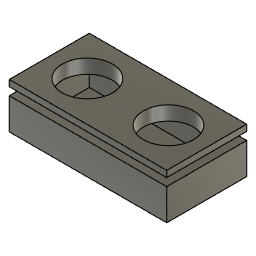
HCSR04 (Autodesk Fusion 360 design; units mm, degrees)
Autodesk Fusion 360 part; units mm, degrees
sketch "top" plane through (0, 0, 0) normal (0, 0, 1) x (1, 0, 0)
  line L0 (22.65, -10.28) -> (-22.65, -10.28)
  line L1 (-22.65, -10.28) -> (-22.65, 10.28)
  line L2 (-22.65, 10.28) -> (22.65, 10.28)
  line L3 (22.65, 10.28) -> (22.65, -10.28)
  line L4 (22.65, -10.28) -> (-22.65, 10.28) construction
  line L5 (-22.65, -10.28) -> (22.65, 10.28) construction
  circle A0 centre (12.95, -0.02) radius 8
  circle A1 centre (-12.95, -0.02) radius 8
  line L6 (-4.95, 0) -> (4.95, 0) construction
  line L7 (-5, -10.28) -> (5, -10.28)
  line L8 (5, -10.28) -> (5, -7.48)
  line L9 (5, -7.48) -> (-5, -7.48)
  line L10 (-5, -7.48) -> (-5, -10.28)
  line L11 (0, -7.48) -> (0, -10.28) construction
  line L12 (25.15, -12.78) -> (-25.15, -12.78)
  line L13 (-25.15, -12.78) -> (-25.15, 12.78)
  line L14 (-25.15, 12.78) -> (25.15, 12.78)
  line L15 (25.15, 12.78) -> (25.15, -12.78)
  line L16 (22.525, -10.155) -> (-22.525, -10.155)
  line L17 (-22.525, -10.155) -> (-22.525, 10.155)
  line L18 (-22.525, 10.155) -> (22.525, 10.155)
  line L19 (22.525, 10.155) -> (22.525, -10.155)
  dimension "d1" = 45.3
  dimension "d2" = 20.56
  dimension "d3" = 16
  dimension "d4" = 16
  dimension "d5" = 2.3
  dimension "d6" = 1.7
  dimension "d7" = 1.7
  dimension "d8" = 2.3
  dimension "d9" = 2.8
  dimension "d10" = 10
  dimension "d11" = -2.5
  dimension "d20" = 0.125
  constraint horizontal L0
  constraint perpendicular L0 L1
  constraint parallel L0 L2
  constraint parallel L1 L3
  constraint coincident L4 origin
  constraint coincident L5 origin
  constraint coincident A1 L6.start
  constraint coincident A0 L6.end
  constraint horizontal L6
  constraint horizontal L7
  constraint vertical L8
  constraint horizontal L9
  constraint vertical L10
  constraint coincident L0 L7.start
  constraint midpoint L9 L11.start
  constraint midpoint L7 L11.end
  constraint midpoint L0 L11.end
  measures "d1" distance of L1.end L2.end
  measures "d2" distance of L0.end L1.end
  measures "d3" diameter of A0
  measures "d4" diameter of A1
  measures "d5" distance of L2 A0
  measures "d6" distance of L3 A0
  measures "d7" distance of L1 A1
  measures "d8" distance of L2 A1
  measures "d9" distance of L7.start L9.end
  measures "d10" distance of L8.end L9.end
extrude "Extrude1" add sketch "top" along normal blind 2 contours L0 L1 L2 L3 L8 L10 L16 L17 L18 L19 | L8 L9 L10 L16 L17 L18 L19 | A0 | A1 | L12 L13 L14 L15 makes body 1
extrude "Extrude2" add sketch "top" along normal blind 8 from surface at 2 contours L12 L13 L14 L15 bodies 1
extrude "Extrude4" add sketch "top" along normal blind 2.5 from surface at 10 separate body contours L8 L9 L10 L16 | L8 L9 L10 L16 L17 L18 L19 makes body 2
extrude "Extrude5" add sketch "top" along normal blind 2 from surface at 12.5 contours L0 L1 L2 L3 L8 L10 L16 L17 L18 L19 | L0 L7 L8 L10 L16 | L8 L9 L10 L16 | L8 L9 L10 L16 L17 L18 L19 | L12 L13 L14 L15 bodies 2
named bodies: "HCSR04-enclosure", "HCSR04-lid"
